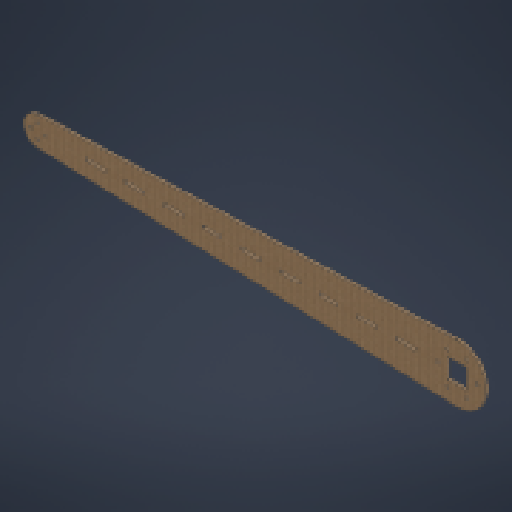
# Autodesk Inventor part: MainArm
Saved by Autodesk Inventor 2024.1 (Build 281209000, 209)
## iProperties
Created: 2023-10-16
Part Number: MainArm
Material: MDF Medium Density Fiberboard
Document SubType Name: Modeling
Designer: Brandon
Density: 0.8 g/cm^3
Appearance: Cardboard - Corrugated
Author: Brandon
Autodesk Inventor part; units mm, degrees
ref_plane "YZ Plane" through (0, 0, 0) normal (1, 0, 0) x (0, 1, 0)
ref_plane "XZ Plane" through (0, 0, 0) normal (0, 1, 0) x (-1, 0, 0)
ref_plane "XY Plane" through (0, 0, 0) normal (0, 0, 1) x (1, 0, 0)
sketch "Sketch1" plane through (0, 0, 0) normal (0, 0, 1) x (1, 0, 0)
  circle A0 centre (0, 0) radius 31.75 projected
  circle A1 centre (25.4, 0) radius 2.1 projected
  circle A2 centre (-25.4, 0) radius 2.1 projected
  circle A3 centre (12.7, -21.997) radius 2.1 projected
  circle A4 centre (-12.7, -21.997) radius 2.1 projected
  line L0 (12.7, -12.7) -> (12.7, 12.7) projected
  line L1 (-12.7, -12.7) -> (12.7, -12.7) projected
  line L2 (-12.7, 12.7) -> (-12.7, -12.7) projected
  line L3 (12.7, 12.7) -> (-12.7, 12.7) projected
  circle A5 centre (12.7, 21.997) radius 2.1 projected
  circle A6 centre (-12.7, 21.997) radius 2.1 projected
  circle A7 centre (0, 0) radius 38.1
  line L4 (0, 0) -> (-550, 0)
  circle A8 centre (-550, 0) radius 19.05
  circle A9 centre (-540.475, 0) radius 2
  circle A10 centre (-550, 9.525) radius 2
  circle A11 centre (-559.525, 0) radius 2
  circle A12 centre (-550, -9.525) radius 2
  line L5 (-1.3196, 38.0771) -> (-550.6598, 19.0386)
  line L6 (-1.3196, -38.0771) -> (-550.6598, -19.0386)
  circle A13 centre (12.7, 21.997) radius 2
  circle A14 centre (-12.7, 21.997) radius 2
  circle A15 centre (25.4, 0) radius 2
  circle A16 centre (-25.4, 0) radius 2
  circle A17 centre (12.7, -21.997) radius 2
  circle A18 centre (-12.7, -21.997) radius 2
  line L7 (-486.5, -1.5875) -> (-461.1, -1.5875)
  line L8 (-461.1, -1.5875) -> (-461.1, 1.5875)
  line L9 (-461.1, 1.5875) -> (-486.5, 1.5875)
  line L10 (-486.5, 1.5875) -> (-486.5, -1.5875)
  line L11 (-410.3, -1.5875) -> (-410.3, 1.5875)
  line L12 (-435.7, -1.5875) -> (-410.3, -1.5875)
  line L13 (-410.3, 1.5875) -> (-435.7, 1.5875)
  line L14 (-435.7, 1.5875) -> (-435.7, -1.5875)
  line L15 (-359.5, -1.5875) -> (-359.5, 1.5875)
  line L16 (-384.9, -1.5875) -> (-359.5, -1.5875)
  line L17 (-359.5, 1.5875) -> (-384.9, 1.5875)
  line L18 (-384.9, 1.5875) -> (-384.9, -1.5875)
  line L19 (-308.7, -1.5875) -> (-308.7, 1.5875)
  line L20 (-334.1, -1.5875) -> (-308.7, -1.5875)
  line L21 (-308.7, 1.5875) -> (-334.1, 1.5875)
  line L22 (-334.1, 1.5875) -> (-334.1, -1.5875)
  line L23 (-257.9, -1.5875) -> (-257.9, 1.5875)
  line L24 (-283.3, -1.5875) -> (-257.9, -1.5875)
  line L25 (-257.9, 1.5875) -> (-283.3, 1.5875)
  line L26 (-283.3, 1.5875) -> (-283.3, -1.5875)
  line L27 (-207.1, -1.5875) -> (-207.1, 1.5875)
  line L28 (-232.5, -1.5875) -> (-207.1, -1.5875)
  line L29 (-207.1, 1.5875) -> (-232.5, 1.5875)
  line L30 (-232.5, 1.5875) -> (-232.5, -1.5875)
  line L31 (-156.3, -1.5875) -> (-156.3, 1.5875)
  line L32 (-181.7, -1.5875) -> (-156.3, -1.5875)
  line L33 (-156.3, 1.5875) -> (-181.7, 1.5875)
  line L34 (-181.7, 1.5875) -> (-181.7, -1.5875)
  line L35 (-105.5, -1.5875) -> (-105.5, 1.5875)
  line L36 (-130.9, -1.5875) -> (-105.5, -1.5875)
  line L37 (-105.5, 1.5875) -> (-130.9, 1.5875)
  line L38 (-130.9, 1.5875) -> (-130.9, -1.5875)
  line L39 (-54.7, -1.5875) -> (-54.7, 1.5875)
  line L40 (-80.1, -1.5875) -> (-54.7, -1.5875)
  line L41 (-54.7, 1.5875) -> (-80.1, 1.5875)
  line L42 (-80.1, 1.5875) -> (-80.1, -1.5875)
  point P0 (-486.5, 0)
  point P1 (-473.8, -1.5875)
  point P2 (-423, -1.5875)
  point P3 (-435.7, 0)
  point P4 (-372.2, -1.5875)
  point P5 (-384.9, 0)
  point P6 (-321.4, -1.5875)
  point P7 (-334.1, 0)
  point P8 (-270.6, -1.5875)
  point P9 (-283.3, 0)
  point P10 (-219.8, -1.5875)
  point P11 (-232.5, 0)
  point P12 (-169, -1.5875)
  point P13 (-181.7, 0)
  point P14 (-118.2, -1.5875)
  point P15 (-130.9, 0)
  point P16 (-67.4, -1.5875)
  point P17 (-80.1, 0)
  dimension "d0" = 76.2
  dimension "d1" = 550
  dimension "d2" = 38.1
  dimension "d3" = 4
  dimension "d4" = 9.525
  dimension "d7" = 360
  dimension "d9" = 4
  dimension "d10" = 4
  dimension "d11" = 4
  dimension "d12" = 4
  dimension "d13" = 4
  dimension "d14" = 4
  dimension "d17" = 25.4
  dimension "d18" = 3.175
  dimension "d19" = 76.2
  dimension "d22" = 50.8
  constraints: 78 end point, 12 centre point, 8 coincident, 4 point on circle, 4 tangent, 3 horizontal, 2 midpoint, 2 parallel, 2 point on line, 1 perpendicular, 89 other
  measures "d0" diameter of A7
  measures "d1" distance of L4.start L4.end
  measures "d2" diameter of A8
  measures "d3" diameter of A9
  measures "d4" distance of L4.end A9.centre
  measures "d9" diameter of A13
  measures "d10" diameter of A14
  measures "d11" diameter of A15
  measures "d12" diameter of A16
  measures "d13" diameter of A17
  measures "d14" diameter of A18
  measures "d17" distance of L9.end L8.end
  measures "d18" distance of L8.end L7.end
  measures "d19" horizontal distance of L4.end point (-473.8, -1.587)
  measures "d22" distance of L8.end L11.end
extrude "Extrusion1" add sketch "Sketch1" along normal blind 3.175 contours A0 | A7 | A7 L6 A8 L4 L10 L7 L8 L14 L12 L11 L18 L16 L15 L22 L20 L19 L26 L24 L23 L30 L28 L27 L34 L32 L31 L38 L36 L35 L42 L40 L39 | L4 L39 L41 L42 L35 L37 L38 L31 L33 L34 L27 L29 L30 L23 L25 L26 L19 L21 L22 L15 L17 L18 L11 L13 L14 L8 L9 L10 A8 L5 A7 | A8
body "Solid1"
